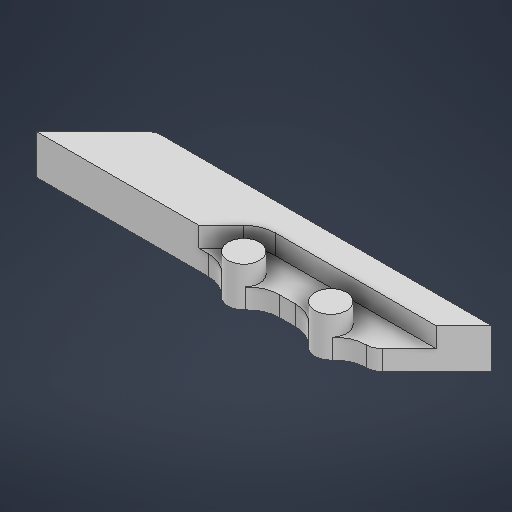
# Autodesk Inventor part: Dispenser
Saved by Autodesk Inventor 2026.2 (Build 302298000, 298)
## iProperties
Created: 2026-03-23
Part Number: Dispenser
Material: Generic
Document SubType Name: Modeling
Designer: Cobble
Density: 1 g/cm^3
Appearance: Default
Author: Cobble
Autodesk Inventor part; units mm, degrees
ref_plane "YZ Plane" through (0, 0, 0) normal (1, 0, 0) x (0, 1, 0)
ref_plane "XZ Plane" through (0, 0, 0) normal (0, 1, 0) x (-1, 0, 0)
ref_plane "XY Plane" through (0, 0, 0) normal (0, 0, 1) x (1, 0, 0)
sketch "Sketch1" plane through (0, 0, 0) normal (0, 0, 1) x (1, 0, 0)
  line L0 (0, 0) -> (140, 0)
  line L1 (140, 0) -> (140, 60) construction
  line L2 (140, 60) -> (0, 60) construction
  line L3 (0, 60) -> (0, 0) construction
  line L4 (0, 45) -> (15, 60)
  line L5 (0, 45) -> (21.2132, 45) construction
  line L6 (0, 45) -> (140, 45) construction
  line L7 (140, 45) -> (125, 60)
  line L8 (140, 45) -> (161.2132, 45) construction
  line L9 (0, 0) -> (0, 45)
  line L10 (140, 0) -> (140, 45)
  line L11 (125, 60) -> (15, 60)
  line L12 (0, 0) -> (140, 0)
  line L13 (140, 0) -> (140, 5)
  line L14 (140, 5) -> (0, 5) construction
  line L15 (0, 5) -> (0, 0)
  line L16 (0, 0) -> (5, 0)
  line L17 (5, 0) -> (5, 50) construction
  line L18 (5, 50) -> (0, 50) construction
  line L19 (0, 50) -> (0, 0) construction
  line L20 (140, 0) -> (135, 0) construction
  line L21 (135, 0) -> (135, 50) construction
  line L22 (135, 50) -> (140, 50) construction
  line L23 (140, 50) -> (140, 0) construction
  line L24 (0, 45) -> (30, 45)
  line L25 (140, 45) -> (30, 45)
  line L26 (85, 45) -> (100, 60)
  line L27 (140, 45) -> (115.9454, 45)
  line L28 (115.9454, 0) -> (140, 0)
  line L29 (140, 0) -> (140, 45)
  line L30 (0, 0) -> (10, 0)
  line L31 (10, 0) -> (10, 45)
  line L32 (10, 45) -> (0, 45)
  line L33 (0, 45) -> (0, 0)
  line L34 (10, 5) -> (77.1751, 5) construction
  circle A0 centre (81.8934, 52.5) radius 7.5 construction
  line L35 (81.8934, 52.5) -> (39.467, 10.0736) construction
  line L36 (81.8934, 52.5) -> (141.8934, 52.5) construction
  circle A1 centre (39.467, 10.0736) radius 7.5 construction
  circle A2 centre (17.5, 10.0736) radius 7.5 construction
  line L37 (17.5, 10.0736) -> (39.467, 10.0736) construction
  line L38 (17.5, 10.0736) -> (59.9264, 52.5) construction
  line L39 (17.5, 10.0736) -> (77.5, 10.0736) construction
  circle A3 centre (59.9264, 52.5) radius 7.5 construction
  line L40 (59.9264, 52.5) -> (81.8934, 52.5) construction
  circle A4 centre (52.4264, 45) radius 7.5 construction
  circle A5 centre (74.3934, 45) radius 7.5 construction
  line L41 (12.1967, 15.3769) -> (47.1231, 50.3033) construction
  line L42 (57.7297, 39.6967) -> (22.8033, 4.7703) construction
  line L43 (34.1637, 15.3769) -> (69.0901, 50.3033) construction
  line L44 (79.6967, 39.6967) -> (44.7703, 4.7703) construction
  circle A6 centre (52.4264, 45) radius 8
  circle A7 centre (74.3934, 45) radius 8
  line L45 (52.4264, 45) -> (74.3934, 45)
  line L46 (46.7696, 50.6569) -> (41.1127, 45)
  line L47 (46.7696, 50.6569) -> (54.7696, 50.6569) construction
  line L48 (80.0503, 50.6569) -> (88.0503, 50.6569) construction
  line L49 (52.4264, 53) -> (93, 53)
  circle A8 centre (52.4264, 45) radius 4
  circle A9 centre (74.3934, 45) radius 4
  point P0 (89, 53)
  point P1 (81, 53)
  point P2 (60.4264, 45)
  point P3 (44.4264, 45)
  point P4 (78.3934, 45)
  point P5 (70.3934, 45)
  dimension "d20" = 16
  dimension "d0" = 140
  dimension "d1" = 60
  dimension "d2" = 45
  dimension "d3" = 15
  dimension "d4" = 135
  dimension "d5" = 5
  dimension "d6" = 5
  dimension "d7" = 5
  dimension "d8" = 25
  dimension "d9" = 10
  dimension "d11" = 60
  dimension "d12" = 135
  dimension "d13" = 15
  dimension "d14" = 15
  dimension "d15" = 60
  dimension "d16" = 45
  dimension "d17" = 15
  dimension "d18" = 15
  dimension "d19" = 16
  dimension "d21" = 135
  dimension "d27" = 8
  dimension "d28" = 8
  constraints: 100 end point, 22 point on line, 16 parallel, 15 horizontal, 12 tangent, 10 point on circle, 9 centre point, 6 coincident, 6 perpendicular, 5 collinear, 5 equal length, 1 midpoint, 3 other
  measures "d0" distance of L2.end L1.end
  measures "d1" distance of L1.end L0.end
  measures "d2" angle of L5 L4
  measures "d3" distance of L2.end L4.start
  measures "d4" angle of L8 L7
  measures "d5" distance of L13.end L12.end
  measures "d6" distance of L18.end L17.end
  measures "d7" distance of L21.end L22.end
  measures "d8" distance of L7.end L26.end
  measures "d9" distance of L32.end L31.end
  measures "d11" distance of L35.start L35.end
  measures "d12" angle of L35 L36
  measures "d13" diameter of A1
  measures "d14" diameter of A2
  measures "d15" distance of L37.start L38.end
  measures "d16" angle of L39 L38
  measures "d17" diameter of A4
  measures "d18" diameter of A5
  measures "d19" diameter of A6
  measures "d21" angle of L46 L47
  measures "d27" diameter of A8
  measures "d28" diameter of A9
extrude "Extrusion1" add sketch "Sketch1" along normal blind 10 contours L4 L11 L26 L49 A6 L46 L25 L24 | A8 L25 | L25 A8 | A9 L25 | L25 A9
extrude "Extrusion2" add sketch "Sketch1" along normal blind 5 contours L46 A6 L25 | L26 L25 A7 L49 | A6 L25 A8 | A7 L25 A9 | A7 L25 A6 L49 | A8 L25 | L25 A9 picked at (59.0262, 45.5934) picked at (80.9932, 45.5934) picked at (49.7985, 45.3191) picked at (71.7655, 45.3191)
fillet "Fillet1" radius 8 4 edges at (48.4264, 45, 2.5) (56.4264, 45, 2.5) (78.3934, 45, 2.5) (70.3934, 45, 2.5)
fillet "Fillet2" radius 4 2 edges at (15, 60, 5) (85, 45, 2.5)
body "Solid1"
